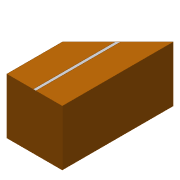
# Autodesk Inventor part: Highland_赤
Saved by Autodesk Inventor 2015 SP1 (Build 190203100, 203)
## iProperties
Created: 2015-08-24
Part Number: Highland_赤
Material: 一般
Document SubType Name: Modeling
Designer: nobuhiro
Density: 1 g/cm^3
Appearance: オレンジ
Author: nobuhiro
Autodesk Inventor part; units mm, degrees
ref_plane "YZ Plane" through (0, 0, 0) normal (1, 0, 0) x (0, 1, 0)
ref_plane "XZ Plane" through (0, 0, 0) normal (0, 1, 0) x (-1, 0, 0)
ref_plane "XY Plane" through (0, 0, 0) normal (0, 0, 1) x (1, 0, 0)
sketch "スケッチ1" plane through (0, 0, 0) normal (0, 0, 1) x (1, 0, 0)
  line L0 (-300, 0) -> (300, 0)
  line L1 (300, 0) -> (300, 600)
  line L2 (300, 600) -> (-300, 600)
  line L3 (-300, 600) -> (-300, 0)
  line L4 (-300, 600) -> (300, 1200)
  line L5 (300, 1200) -> (300, 600)
  point P0 (0, 0)
  point P1 (0, 0)
  dimension "d0" = 45
  dimension "d1" = 600
  dimension "d2" = 600
  constraints: 12 end point, 2 coincident, 2 parallel, 1 horizontal, 1 midpoint, 1 perpendicular, 1 vertical
  measures "d0" angle of L4 L2
  measures "d1" distance between parallel lines of L0 L2
  measures "d2" distance between parallel lines of L1 L3
extrude "押し出し1" add sketch "スケッチ1" along normal blind 600
sketch "スケッチ2" plane through (0, 0, 600) normal (0, 0, 1) x (1, 0, 0)
  line L0 (300, 1200) -> (-300, 600) projected
  line L1 (-300, 0) -> (300, 0) projected
  line L2 (-15, 0) -> (15, 0)
  line L3 (15, 0) -> (15, 915)
  line L4 (15, 915) -> (-15, 885)
  line L5 (-15, 885) -> (-15, 0)
  point P0 (0, 0)
  point P1 (0, 0)
  point P2 (0, 0)
  dimension "d5" = 30
  constraints: 8 end point, 3 point on line, 2 midpoint, 1 coincident, 1 horizontal, 1 parallel, 1 perpendicular
  measures "d5" distance between parallel lines of L3 L5
extrude "押し出し2" add sketch "スケッチ2" along normal blind 0.1
